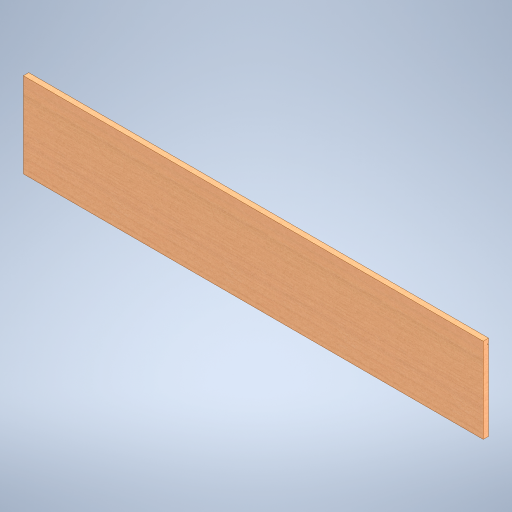
# Autodesk Inventor part: Längsseite_Gehäuse
Saved by Autodesk Inventor 2024 (Build 280153000, 153)
## iProperties
Created: 2024-03-12
Part Number: Längsseite_Gehäuse
Material: Holz (Kirsche)
Document SubType Name: Modeling
Designer: haniv
Density: 0.63 g/cm^3
Appearance: Kirsche - natur - schwacher Glanz
Author: haniv
Autodesk Inventor part; units mm, degrees
ref_plane "YZ Plane" through (0, 0, 0) normal (1, 0, 0) x (0, 1, 0)
ref_plane "XZ Plane" through (0, 0, 0) normal (0, 1, 0) x (-1, 0, 0)
ref_plane "XY Plane" through (0, 0, 0) normal (0, 0, 1) x (1, 0, 0)
sketch "Skizze1" plane through (0, 0, 0) normal (0, 1, 0) x (-1, 0, 0)
  line L0 (-514, 95) -> (514, 95)
  line L1 (514, 95) -> (514, -95)
  line L2 (514, -95) -> (-514, -95)
  line L3 (-514, -95) -> (-514, 95)
  point P0 (0, 0)
  point P1 (0, 95)
  point P2 (514, 0)
  dimension "d0" = 1028
  dimension "d1" = 190
  constraints: 8 end point, 2 midpoint, 2 parallel, 1 horizontal, 1 horizontal alignment, 1 perpendicular, 1 vertical alignment
  measures "d0" distance of L1.end L2.end
  measures "d1" distance of L2.end L0.start
extrude "Extrusion1" add sketch "Skizze1" along normal blind 12
sketch "Skizze2" plane through (0, 12, 0) normal (0, 1, 0) x (1, 0, 0)
  line L0 (514, 95) -> (-514, 95) projected
  line L1 (-514, 95) -> (-514, -95) projected
  line L2 (-514, -95) -> (514, -95) projected
  line L3 (514, -95) -> (514, 95) projected
  line L4 (-514, -85) -> (514, -85)
  line L5 (514, -85) -> (514, -82.8)
  line L6 (514, -82.8) -> (-514, -82.8)
  line L7 (-514, -82.8) -> (-514, -85)
  point P0 (0, 0)
  dimension "d4" = 2.2
  dimension "d5" = 10
  constraints: 8 end point, 2 parallel, 2 point on line, 1 horizontal, 1 perpendicular
  measures "d4" distance between parallel lines of L6 L4
  measures "d5" distance between parallel lines of L2 L4
extrude "Extrusion2" cut sketch "Skizze2" against normal blind 2.2 contours L3 L4 L1 L6
equation "\"d6\" = d4"
